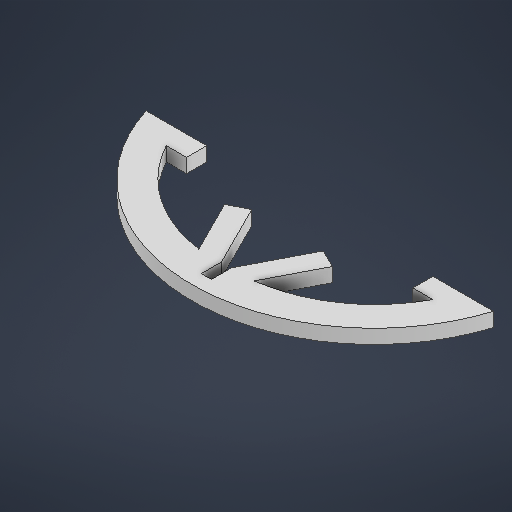
# Autodesk Inventor part: Droplet Launcher 2
Saved by Autodesk Inventor 2026.1 (Build 301233020, 233B)
## iProperties
Created: 2026-02-02
Part Number: Droplet Launcher 2
Material: Generic
Document SubType Name: Modeling
Designer: jacob
Density: 1 g/cm^3
Appearance: Default
Author: jacob
Autodesk Inventor part; units mm, degrees
ref_plane "YZ Plane" through (0, 0, 0) normal (1, 0, 0) x (0, 1, 0)
ref_plane "XZ Plane" through (0, 0, 0) normal (0, 1, 0) x (-1, 0, 0)
ref_plane "XY Plane" through (0, 0, 0) normal (0, 0, 1) x (1, 0, 0)
sketch "Sketch1" plane through (0, 0, 0) normal (0, 1, 0) x (-1, 0, 0)
  line L0 (86.0424, 26.9023) -> (56.0424, 26.9023)
  line L1 (2.5, 83.15) -> (-2.5, 83.15)
  line L2 (2.5, 83.15) -> (2.5, 73.15)
  line L3 (-2.5, 83.15) -> (-2.5, 73.15)
  circle A0 centre (0, 0) radius 90.15
  line L4 (-86.0424, 26.9023) -> (-56.0424, 26.9023)
  line L5 (-56.0424, 26.9023) -> (-56.0424, 36.9023)
  line L6 (-56.0424, 36.9023) -> (-66.0424, 36.9023)
  line L7 (56.0424, 26.9023) -> (56.0424, 36.9023)
  line L8 (56.0424, 36.9023) -> (66.0424, 36.9023)
  line L9 (-17.9658, 43.15) -> (-2.5, 73.15)
  line L10 (17.5, 43.15) -> (2.5, 73.15)
  line L11 (17.5, 43.15) -> (26.4443, 47.6221)
  line L12 (26.4443, 47.6221) -> (13.6803, 73.15)
  line L13 (-17.9658, 43.15) -> (-26.9101, 47.6221)
  line L14 (-26.9101, 47.6221) -> (-13.7498, 73.15)
  arc A1 (66.0424, 36.9023) -> (13.6803, 73.15) centre (4.3796, 3.7706) ccw
  arc A2 (-13.7498, 73.15) -> (-66.0424, 36.9023) centre (-4.3742, 3.7807) ccw
  dimension "d28" = 180.3
  dimension "d1" = 30
  dimension "d20" = 5
  dimension "d21" = 10
  dimension "d22" = 10
  dimension "d29" = 30
  dimension "d30" = 10
  dimension "d31" = 10
  dimension "d32" = 10
  dimension "d33" = 10
  dimension "d37" = 10
  dimension "d38" = 10
  dimension "d39" = 70
  dimension "d40" = 70
  constraints: 30 end point, 4 perpendicular, 4 point on circle, 3 vertical, 2 centre point, 2 horizontal, 1 coincident, 1 parallel, 1 point on line, 3 other
  measures "d1" distance of L0.start L0.end
  measures "d20" distance of L1.start L1.end
  measures "d21" distance of L1.start L2.end
  measures "d22" distance of L1.end L3.end
  measures "d29" distance of L4.start L4.end
  measures "d30" distance of L4.end L5.end
  measures "d31" distance of L5.end L6.end
  measures "d32" distance of L0.end L7.end
  measures "d33" distance of L7.end L8.end
  measures "d37" distance of L10.start L11.end
  measures "d38" distance of L9.start L13.end
  measures "d39" radius of A1
  measures "d40" radius of A2
extrude "Extrusion1" add sketch "Sketch1" along normal blind 7 contours L0 L7 L8 A1 L12 L11 L10 L2 L1 L3 L9 L13 L14 A2 L6 L5 L4 A0 picked at (-11.4052, 63.15)
sketch "Sketch2" plane through (0, 0, 0) normal (0, -1, 0) x (1, 0, 0)
  circle A0 centre (74.2273, 36.5899) radius 3.35
  circle A1 centre (-74.0777, 36.5899) radius 3.35
  circle A2 centre (-13.319, 81.4854) radius 3.35
  circle A3 centre (13.1694, 81.4854) radius 3.35
  point P0 (0, 0)
  dimension "d43" = 6.7
  dimension "d44" = 6.7
  dimension "d45" = 6.7
  dimension "d46" = 6.7
  constraints: 4 centre point
  measures "d43" diameter of A0
  measures "d44" diameter of A1
  measures "d45" diameter of A2
  measures "d46" diameter of A3
extrude "Extrusion2" cut sketch "Sketch2" against normal blind 4.7
body "Solid1"
